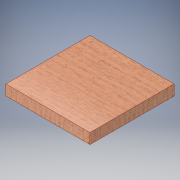
# Autodesk Inventor part: Base
Saved by Autodesk Inventor 2017 (Build 210142000, 142)
## iProperties
Created: 2018-03-09
Part Number: Base
Material: Generic
Document SubType Name: Modeling
Designer: Russ
Density: 1 g/cm^3
Appearance: White Oak - Natural Medium Gloss
Author: Russ
Autodesk Inventor part; units mm, degrees
ref_plane "YZ Plane" through (0, 0, 0) normal (1, 0, 0) x (0, 1, 0)
ref_plane "XZ Plane" through (0, 0, 0) normal (0, 1, 0) x (-1, 0, 0)
ref_plane "XY Plane" through (0, 0, 0) normal (0, 0, 1) x (1, 0, 0)
sketch "Sketch1" plane through (0, 0, 0) normal (0, 1, 0) x (-1, 0, 0)
  line L0 (0, 0) -> (152.4, 0)
  line L1 (152.4, 0) -> (152.4, -152.4)
  line L2 (152.4, -152.4) -> (0, -152.4)
  line L3 (0, -152.4) -> (0, 0)
  dimension "d0" = 152.4
  dimension "d1" = 152.4
  constraints: 8 end point, 2 parallel, 1 horizontal, 1 perpendicular
  measures "d0" distance of L2.end L0.start
  measures "d1" distance of L0.start L0.end
extrude "Extrusion1" add sketch "Sketch1" along normal blind 19.05
body "Solid1"
